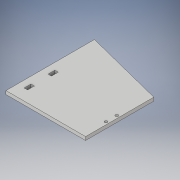
# Autodesk Inventor part: pinball-case-left-wall-outer-scaled
Saved by Autodesk Inventor 2017 (Build 210142000, 142)
## iProperties
Created: 2017-02-27
Part Number: pinball-case-left-wall-outer-scaled
Material: Generic
Document SubType Name: Modeling
Designer: John
Density: 1 g/cm^3
Appearance: Default
Author: John
Autodesk Inventor part; units mm, degrees
ref_plane "YZ Plane" through (0, 0, 0) normal (1, 0, 0) x (0, 1, 0)
ref_plane "XZ Plane" through (0, 0, 0) normal (0, 1, 0) x (-1, 0, 0)
ref_plane "XY Plane" through (0, 0, 0) normal (0, 0, 1) x (1, 0, 0)
sketch "Sketch1" plane through (0, 0, 0) normal (0, 1, 0) x (-1, 0, 0)
  line L0 (0, 0) -> (-70, 0)
  line L1 (-70, 0) -> (-70, -60)
  line L2 (-70, -60) -> (0, -60)
  line L3 (0, -60) -> (0, 0)
  line L4 (0, -60) -> (0, -77.7966)
  line L5 (0, -77.7966) -> (-70, -60)
  dimension "d0" = 70
  dimension "d1" = 60
  dimension "d23" = 14.264
  constraints: 12 end point, 2 parallel, 1 horizontal, 1 perpendicular, 1 vertical
  measures "d0" distance of L2.end L1.end
  measures "d1" distance of L1.end L0.end
  measures "d23" angle of L2 L5
extrude "Extrusion1" add sketch "Sketch1" along normal blind 3
sketch "Sketch3" plane through (0, 3, 0) normal (0, 1, 0) x (1, 0, 0)
  circle A0 centre (67.75, 20.25) radius 1.25
  circle A1 centre (67.75, 29.75) radius 1.25
  line L0 (70, 0) -> (70, 60) projected
  line L1 (0, 0) -> (70, 0) projected
  line L2 (6, 10) -> (9, 10)
  line L3 (9, 10) -> (9, 16)
  line L4 (9, 16) -> (6, 16)
  line L5 (6, 16) -> (6, 10)
  line L6 (6, 37) -> (9, 37)
  line L7 (9, 37) -> (9, 31)
  line L8 (9, 31) -> (6, 31)
  line L9 (6, 31) -> (6, 37)
  line L10 (0, 77.7966) -> (0, 0) projected
  dimension "d15" = 2.5
  dimension "d16" = 2.25
  dimension "d17" = 2.25
  dimension "d18" = 2.5
  dimension "d19" = 20.25
  dimension "d20" = 9.5
  dimension "d24" = 3
  dimension "d25" = 6
  dimension "d26" = 6
  dimension "d27" = 10
  dimension "d28" = 15
  dimension "d29" = 6
  constraints: 16 end point, 4 parallel, 2 centre point, 2 horizontal, 2 perpendicular, 2 point on line
  measures "d15" diameter of A0
  measures "d16" distance from line of L0 A1.centre
  measures "d17" distance from line of L0 A0.centre
  measures "d18" diameter of A1
  measures "d19" distance from line of L1 A0.centre
  measures "d20" distance of A1.centre A0.centre
  measures "d24" distance of L4.end L3.end
  measures "d25" distance of L3.end L2.end
  measures "d26" distance of L6.end L7.end
  measures "d27" distance between parallel lines of L1 L2
  measures "d28" distance between parallel lines of L8 L4
  measures "d29" distance between parallel lines of L10 L5
extrude "Extrusion3" cut sketch "Sketch3" along normal through all both and the other way through all
equation "\"d17\" = d16"
equation "\"d18\" = d15"
body "Solid1"
